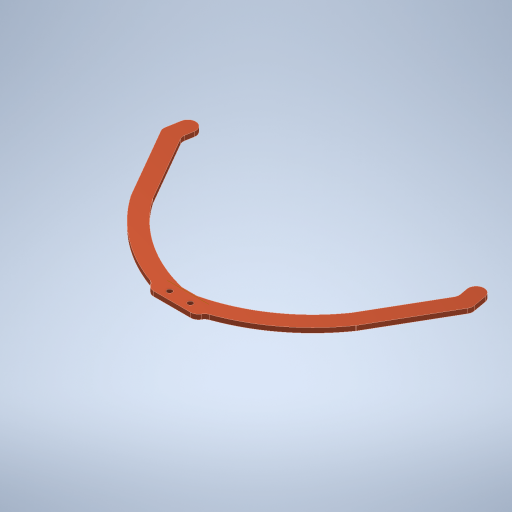
# Autodesk Inventor part: Claw1
Saved by Autodesk Inventor 2023 (Build 270158000, 158)
## iProperties
Created: 2022-11-29
Part Number: Claw1
Material: Copper, Cast
Document SubType Name: Modeling
Designer: kakik
Density: 8.94 g/cm^3
Appearance: Copper - Satin
Author: kakik
Autodesk Inventor part; units mm, degrees
ref_plane "YZ Plane" through (0, 0, 0) normal (1, 0, 0) x (0, 1, 0)
ref_plane "XZ Plane" through (0, 0, 0) normal (0, 1, 0) x (-1, 0, 0)
ref_plane "XY Plane" through (0, 0, 0) normal (0, 0, 1) x (1, 0, 0)
sketch "Sketch1" plane through (0, 0, 0) normal (0, 1, 0) x (-1, 0, 0)
  line L0 (0, 0) -> (0, 10)
  line L1 (0, 10) -> (42.1132, 10)
  line L2 (0, 0) -> (36.3397, 0)
  line L3 (40.6699, -2.5) -> (86.3115, -81.5535)
  line L4 (86.9054, -84.9218) -> (86.0202, -89.942)
  line L5 (90.076, -95.7343) -> (90.076, -95.7343)
  line L6 (95.8682, -91.6785) -> (97.3855, -83.0739)
  line L7 (96.7916, -79.7056) -> (46.4434, 7.5)
  arc A0 (45.5774, 9) -> (43.8453, 10) centre (43.8453, 8) ccw
  arc A1 (40.6699, -2.5) -> (36.3397, 0) centre (36.3397, -5) ccw
  arc A2 (86.9054, -84.9218) -> (86.3115, -81.5535) centre (81.9813, -84.0535) ccw
  arc A3 (97.3855, -83.0739) -> (96.7916, -79.7056) centre (92.4614, -82.2056) ccw
  arc A4 (46.4434, 7.5) -> (42.1132, 10) centre (42.1132, 5) ccw
  arc A5 (90.076, -95.7343) -> (95.8682, -91.6785) centre (90.9442, -90.8103) ccw
  arc A6 (86.0202, -89.942) -> (90.076, -95.7343) centre (90.9442, -90.8103) ccw
  point P0 (85.1519, -94.8661)
  point P1 (95, -96.6025)
  point P2 (45, 10)
  point P3 (90.076, -95.7343)
  dimension "d1" = 120
  dimension "d2" = 140
  dimension "d3" = 45
  dimension "d4" = 50
  dimension "d5" = 10
  dimension "d6" = 10
  dimension "d7" = 10
  dimension "d8" = 2
  dimension "d9" = 5
  constraints: 16 end point, 14 point on circle, 14 tangent, 10 point on line, 7 centre point, 5 equal radius, 3 perpendicular, 1 horizontal, 1 parallel, 1 vertical
  measures "d1" angle of L2 L3
  measures "d2" angle of L3 L4
  measures "d3" distance of L0.end point (45, 10)
  measures "d4" horizontal distance of point (45, 10) point (95, -96.603)
  measures "d5" distance of point (85.152, -94.866) point (95, -96.603)
  measures "d6" distance of L0.start L0.end
  measures "d7" distance between parallel lines of L3 L7
  measures "d8" radius of A0
  measures "d9" radius of A1
extrude "Extrusion1" add sketch "Sketch1" along normal blind 3
sketch "Sketch2" plane through (0, 3, 0) normal (0, 1, 0) x (1, 0, 0)
  line L0 (0, -10) -> (0, 0) projected
  line L1 (0, -5) -> (-25.3234, -5) construction
  point P0 (-6.55, -5)
  dimension "d19" = 6.55
  constraints: 2 end point, 1 horizontal, 1 midpoint, 1 point on line
  measures "d19" distance from line of L0 point (-6.55, -5)
hole "Hole1" at (-6.55, 3, 5) direction (0, -1, 0) diameter 3.2 end through all clearance for "Countersunk Flat Head Screw DIN EN ISO 2009" size "M3" standard "DIN"
mirror "Mirror1" about plane through (0, 0, 0) normal (1, 0, 0) of "Extrusion1", "Hole1"
sketch "Sketch3" plane through (0, 3, 0) normal (0, 1, 0) x (1, 0, 0)
  line L0 (-40.6699, 2.5) -> (-86.3115, 81.5535) projected
  line L1 (-36.3397, 0) -> (36.3397, 0) projected
  arc A0 (-71.1338, 55.2651) -> (0, 0) centre (18.4247, 97.1272) ccw
  line L2 (-40.6699, 2.5) -> (-86.3115, 81.5535) projected
  arc A1 (-40.6699, 2.5) -> (-36.3397, 0) centre (-36.3397, 5) ccw projected
  point P0 (-62.6082, 40.4983)
  constraints: 2 point on circle, 1 centre point, 1 point on line
extrude "Extrusion2" add sketch "Sketch3" against normal up to surface (3 mm away) contours L0 A0 L1 A1
mirror "Mirror2" about plane through (0, 0, 0) normal (1, 0, 0) of "Extrusion2"
fillet "Fillet1" radius 5 1 edges at (0, 1.5, 0)
sketch "Sketch4" plane through (0, 3, 0) normal (0, 1, 0) x (1, 0, 0)
  arc A0 (-62.6082, 40.4983) -> (-0.9815, 0.1913) centre (18.4247, 97.1272) ccw projected
  arc A1 (-70.805, 34.7701) -> (-2.9445, -9.6141) centre (18.4247, 97.1272) ccw
  line L0 (-96.7916, 79.7056) -> (-46.4434, -7.5) projected
  arc A2 (-46.4434, -7.5) -> (-42.1132, -10) centre (-42.1132, -5) ccw projected
  line L1 (-42.1132, -10) -> (42.1132, -10) projected
  line L2 (-16.55, -5.9607) -> (-16.55, -10)
  circle A3 centre (-6.55, -5) radius 1.6 projected
  line L3 (-70.805, 34.7701) -> (-71.0577, 35.1332)
  point P0 (0, 0)
  point P1 (-16.55, -7.9804)
  dimension "d23" = 10
  dimension "d24" = 10
  constraints: 4 end point, 3 point on circle, 2 point on line, 1 centre point, 1 midpoint, 1 perpendicular
  measures "d23" radial gap between concentric circles of A0 A1
  measures "d24" horizontal distance of A3.centre point (-16.55, -7.98)
extrude "Extrusion3" cut sketch "Sketch4" against normal blind 10 contours A1 L2 L1 A2 L0 L3
fillet "Fillet2" radius 5 2 edges at (-16.55, 1.5, 5.9607) (-16.55, 1.5, 10)
mirror "Mirror3" about plane through (0, 0, 0) normal (1, 0, 0) of "Fillet2", "Extrusion3"
ref_plane "Work Plane1" through (-11.6432, 0, 0) normal (0, 0, 1) x (1, 0, 0)
sketch "Sketch5" plane through (-11.6432, 0, 0) normal (0, 0, 1) x (1, 0, 0)
  line L0 (0, 3) -> (23.2863, 3) projected
  line L1 (11.6432, 3) -> (11.6432, 0)
  line L2 (19.7932, 0) -> (16.5932, 0) projected
  line L3 (6.6932, 3) -> (16.5932, 3)
  line L4 (16.5932, 3) -> (16.5932, 0)
  line L5 (16.5932, 0) -> (6.6932, 0)
  line L6 (6.6932, 0) -> (6.6932, 3)
  line L7 (6.6932, 3) -> (16.5932, 0) construction
  line L8 (16.5932, 3) -> (6.6932, 0) construction
  point P0 (11.6432, 1.5)
  constraints: 14 end point, 4 midpoint, 2 parallel, 1 horizontal, 1 perpendicular, 1 vertical
extrude "Extrusion4" add sketch "Sketch5" against normal blind 1
fillet "Fillet3" radius 5 2 edges at (-4.6561, 1.5, -1) (4.6561, 1.5, -1)
body "Solid1"
